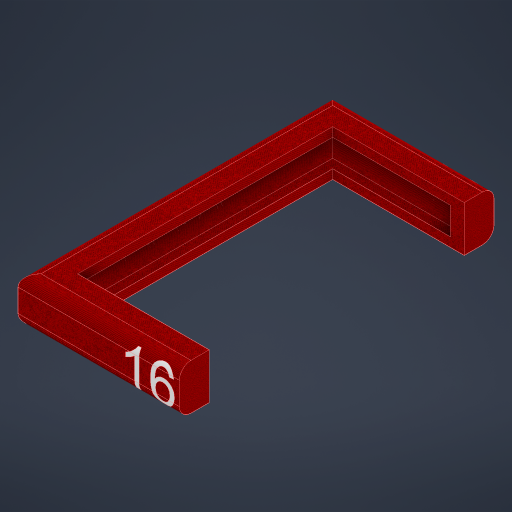
# Autodesk Inventor part: BUMP_005_BumperCloth
Saved by Autodesk Inventor 2024.2 (Build 282272000, 272)
## iProperties
Created: 2024-08-07
Part Number: BUMP_005_BumperCloth
Material: 1000 Denier Nylon Cordura
Document SubType Name: Modeling
Designer: Bryan
Density: 1 g/cm^3
Appearance: Default(1)
Mass: 229.5 g
Surface Area: 11381.8 cm^2
Volume: 229.5 cm^3
Author: Bryan
Autodesk Inventor part; units mm, degrees
ref_plane "YZ Plane" through (0, 0, 0) normal (1, 0, 0) x (0, 1, 0)
ref_plane "XZ Plane" through (0, 0, 0) normal (0, 1, 0) x (-1, 0, 0)
ref_plane "XY Plane" through (0, 0, 0) normal (0, 0, 1) x (1, 0, 0)
sketch "Sketch2" plane through (0, 0, 0) normal (1, 0, 0) x (0, 1, 0)
  line L0 (127, 0) -> (127, -82.55) construction
  line L1 (127, -82.55) -> (0, -82.55) construction
  line L2 (0, -82.55) -> (0, 0) construction
  circle A0 centre (95.25, -50.8) radius 31.75 construction
  circle A1 centre (31.75, -50.8) radius 31.75 construction
  arc A2 (95.25, -82.55) -> (127, -50.8) centre (95.25, -50.8) ccw
  arc A3 (0, -50.8) -> (31.75, -82.55) centre (31.75, -50.8) ccw
  line L3 (31.75, -82.55) -> (95.25, -82.55)
  line L4 (0, -50.8) -> (0, 0)
  line L5 (127, -50.8) -> (127, 0)
  line L6 (127, 0) -> (101.6, 0)
  line L7 (0, 0) -> (25.4, 0)
  line L8 (101.6, 0.4) -> (127.4, 0.4)
  line L9 (127.4, 0.4) -> (127.4, -50.8)
  arc A4 (95.25, -82.95) -> (127.4, -50.8) centre (95.25, -50.8) ccw
  line L10 (95.25, -82.95) -> (31.75, -82.95)
  arc A5 (-0.4, -50.8) -> (31.75, -82.95) centre (31.75, -50.8) ccw
  line L11 (-0.4, -50.8) -> (-0.4, 0.4)
  line L12 (-0.4, 0.4) -> (25.4, 0.4)
  line L13 (127, 0) -> (0, -82.55) construction
  line L14 (0, 0) -> (127, -82.55) construction
  line L15 (101.6, 0.4) -> (101.6, 0)
  line L16 (25.4, 0.4) -> (25.4, 0)
  point P0 (63.5, -41.275)
  dimension "d1" = 82.55
  dimension "d2" = 127
  dimension "d3" = 63.5
  dimension "d4" = 25.4
  dimension "d5" = 25.4
  dimension "d6" = 127
  dimension "d7" = 0.4
  constraints: 34 end point, 12 point on circle, 7 tangent, 6 centre point, 4 point on line, 4 vertical, 3 concentric, 3 horizontal, 1 equal radius, 1 midpoint, 1 parallel, 6 other
  measures "d1" distance of L0.start L0.end
  measures "d2" distance of L2.end L0.start
  measures "d3" diameter of A0
  measures "d4" distance of L0.start L6.end
  measures "d5" distance of L2.end L7.end
  measures "d6" distance of L0.end L1.end
  measures "d7" distance between parallel lines of L6 L8
sketch3d "3D Sketch1"
  line L0 (0, 63.5, -41.275) -> (-407.9875, 63.5, -41.275)
  line L1 (-407.9875, 63.5, -41.275) -> (-407.9875, 63.5, 752.475)
  line L2 (-407.9875, 63.5, 752.475) -> (0, 63.5, 752.475)
  dimension "d10" = 407.9875
  dimension "d11" = 793.75
sweep "Sweep1" add profiles "Sketch2" path "3D Sketch1"
sketch "Sketch3" plane through (0, 31.75, 793.75) normal (1, 0, 0) x (0, 0, -1)
  line L0 (793.75, -31.75) -> (793.75, -6.35) projected
  line L1 (793.75, -6.35) -> (793.35, -6.35) projected
  line L2 (793.35, -6.35) -> (793.35, -32.15) projected
  line L3 (793.35, -32.15) -> (844.55, -32.15) projected
  arc A0 (844.55, -32.15) -> (876.7, 0) centre (844.55, 0) ccw projected
  line L4 (876.7, 0) -> (876.7, 63.5) projected
  arc A1 (876.7, 63.5) -> (844.55, 95.65) centre (844.55, 63.5) ccw projected
  line L5 (844.55, 95.65) -> (793.35, 95.65) projected
  line L6 (793.35, 95.65) -> (793.35, 69.85) projected
  line L7 (793.35, 69.85) -> (793.75, 69.85) projected
  line L8 (793.75, 69.85) -> (793.75, 95.25) projected
  line L9 (793.75, 95.25) -> (844.55, 95.25) projected
  arc A2 (876.3, 63.5) -> (844.55, 95.25) centre (844.55, 63.5) ccw projected
  line L10 (876.3, 63.5) -> (876.3, 0) projected
  arc A3 (844.55, -31.75) -> (876.3, 0) centre (844.55, 0) ccw projected
  line L11 (844.55, -31.75) -> (793.75, -31.75) projected
  line L12 (793.35, 69.85) -> (793.35, -6.35)
  line L13 (82.55, -6.35) -> (82.55, -31.75) projected
  line L14 (82.55, -31.75) -> (31.75, -31.75) projected
  arc A4 (0, 0) -> (31.75, -31.75) centre (31.75, 0) ccw projected
  line L15 (0, 0) -> (0, 63.5) projected
  arc A5 (31.75, 95.25) -> (0, 63.5) centre (31.75, 63.5) ccw projected
  line L16 (31.75, 95.25) -> (82.55, 95.25) projected
  line L17 (82.55, 95.25) -> (82.55, 69.85) projected
  line L18 (82.55, 69.85) -> (82.95, 69.85) projected
  line L19 (82.95, 69.85) -> (82.95, 95.65) projected
  line L20 (82.95, 95.65) -> (31.75, 95.65) projected
  arc A6 (31.75, 95.65) -> (-0.4, 63.5) centre (31.75, 63.5) ccw projected
  line L21 (-0.4, 63.5) -> (-0.4, 0) projected
  arc A7 (-0.4, 0) -> (31.75, -32.15) centre (31.75, 0) ccw projected
  line L22 (31.75, -32.15) -> (82.95, -32.15) projected
  line L23 (82.95, -32.15) -> (82.95, -6.35) projected
  line L24 (82.95, -6.35) -> (82.55, -6.35) projected
  line L25 (82.95, 69.85) -> (82.95, -6.35)
  constraints: 4 end point, 2 vertical
extrude "Extrusion1" add sketch "Sketch3" along normal blind 0.4
sketch "Sketch4" plane through (-366.3125, 101.6, 710.8) normal (0, 0, -1) x (-1, 0, 0)
  line L0 (0, 0) -> (-366.3125, 0) projected
  line L1 (-366.3125, -76.2) -> (-366.3125, 0) projected
  line L2 (0, -76.2) -> (-366.3125, -76.2) projected
  line L3 (-328.2125, 0) -> (-328.2125, -76.2)
  point P0 (-366.3125, -101.6)
  dimension "d16" = 38.1
  constraints: 2 end point, 2 point on line, 1 vertical
  measures "d16" distance between parallel lines of L1 L3
extrude "Extrusion2" add sketch "Sketch4" against normal blind 0.4
sketch "Sketch6" plane through (0, 31.75, 793.75) normal (1, 0, 0) x (0, 0, -1)
  line L0 (82.95, 95.65) -> (31.75, 95.65) projected
  arc A0 (31.75, 95.65) -> (-0.4, 63.5) centre (31.75, 63.5) ccw construction
  line L1 (-0.4, 63.5) -> (-0.4, 0) projected
  arc A1 (-0.4, 0) -> (31.75, -32.15) centre (31.75, 0) ccw projected
  line L2 (31.75, -32.15) -> (82.95, -32.15) projected
  line L3 (82.95, -32.15) -> (82.95, 95.65) projected
  arc A2 (31.75, 95.75) -> (-0.5, 63.5) centre (31.75, 63.5) ccw
  line L4 (31.75, 95.75) -> (83.05, 95.75)
  line L5 (83.05, 95.75) -> (83.05, -32.25)
  line L6 (83.05, -32.25) -> (31.75, -32.25)
  arc A3 (-0.5, 0) -> (31.75, -32.25) centre (31.75, 0) ccw
  line L7 (-0.5, 0) -> (-0.5, 63.5)
  arc A4 (31.75, 146.55) -> (-51.3, 63.5) centre (31.75, 63.5) ccw
  line L8 (31.75, 146.55) -> (133.85, 146.55)
  line L9 (133.85, 146.55) -> (133.85, -83.05)
  line L10 (133.85, -83.05) -> (31.75, -83.05)
  arc A5 (-51.3, 0) -> (31.75, -83.05) centre (31.75, 0) ccw
  line L11 (-51.3, 0) -> (-51.3, 63.5)
  point P0 (793.75, -31.75)
  dimension "d22" = 0.1
  dimension "d51" = 50.8
  constraints: 16 end point, 8 point on circle, 4 centre point, 10 other
  measures "d22" radial gap between concentric circles of A0 A2
  measures "d51" radial gap between concentric circles of A2 A4
ref_plane "Work Plane1" through (-449.6625, 31.75, 794.25) normal (0, 0, 1) x (1, 0, 0)
sketch "Sketch5" plane through (-366.3125, -0.4, 0.4) normal (0, 0, 1) x (1, 0, 0)
  line L0 (366.3125, 102) -> (0, 102) projected
  line L1 (366.3125, 102) -> (366.3125, 25.8) projected
  line L2 (366.3125, 25.8) -> (0, 25.8) projected
  line L3 (328.2125, 102) -> (328.2125, 25.8)
  point P0 (366.3125, 0.4)
  dimension "d19" = 38.1
  constraints: 2 end point, 2 point on line, 1 vertical
  measures "d19" distance between parallel lines of L1 L3
extrude "Extrusion3" add sketch "Sketch5" against normal blind 0.4
sketch "Sketch9" plane through (-449.6625, 31.75, 794.25) normal (0, 0, 1) x (1, 0, 0)
  line L0 (284.9625, 82.95) -> (437.3625, 82.95) construction
  line L1 (437.3625, 82.95) -> (437.3625, -18.65) construction
  line L2 (437.3625, -18.65) -> (284.9625, -18.65) construction
  line L3 (284.9625, -18.65) -> (284.9625, 82.95) construction
  line L4 (32.15, 95.65) -> (450.0625, 95.65) projected
  line L5 (450.0625, 63.5) -> (450.0625, 0) projected
  line L6 (337.7759, -19.0372) -> (325.3082, -19.0372)
  line L7 (325.3082, -19.0372) -> (325.3082, 60.4152)
  spline S0 degree 2 poles (325.3082, 60.4152) (320.8168, 56.1561) (306.1808, 47.5604) (300.3729, 45.3921) knots 0 0 0 1 2 2 2
  line L8 (300.3729, 45.3921) -> (300.3729, 57.4726)
  spline S1 degree 2 poles (300.3729, 57.4726) (310.8271, 62.3512) (326.4698, 76.3677) (329.7223, 82.95) knots 0 0 0 1 2 2 2
  line L9 (329.7223, 82.95) -> (337.7759, 82.95)
  line L10 (337.7759, 82.95) -> (337.7759, -19.0372)
  line L11 (434.5747, 57.6274) -> (422.1844, 56.6207)
  spline S2 degree 2 poles (422.1844, 56.6207) (420.4808, 63.9774) (417.4607, 67.3848) knots 0 0 0 1 1 1
  spline S3 degree 2 poles (417.4607, 67.3848) (412.3497, 72.728) (404.9155, 72.728) knots 0 0 0 1 1 1
  spline S4 degree 2 poles (404.9155, 72.728) (398.9527, 72.728) (394.4613, 69.3982) knots 0 0 0 1 1 1
  spline S5 degree 2 poles (394.4613, 69.3982) (388.5759, 65.139) (381.7613, 48.5671) (381.6064, 33.3116) knots 0 0 0 1 2 2 2
  spline S6 degree 2 poles (381.6064, 33.3116) (386.0979, 40.2037) (399.1851, 46.8634) (406.3094, 46.8634) knots 0 0 0 1 2 2 2
  spline S7 degree 2 poles (406.3094, 46.8634) (418.7771, 46.8634) (436.3558, 28.5104) (436.3558, 13.9518) knots 0 0 0 1 2 2 2
  spline S8 degree 2 poles (436.3558, 13.9518) (436.3558, 4.4268) (428.0698, -11.9902) (413.6662, -20.7409) (404.5284, -20.7409) knots 0 0 0 1 2 3 3 3
  spline S9 degree 2 poles (404.5284, -20.7409) (388.8857, -20.7409) (369.2162, 2.1811) (369.2162, 28.5104) knots 0 0 0 1 2 2 2
  spline S10 degree 2 poles (369.2162, 28.5104) (369.2162, 57.9372) (380.1351, 71.3341) knots 0 0 0 1 1 1
  spline S11 degree 2 poles (380.1351, 71.3341) (389.5826, 82.95) (405.6899, 82.95) knots 0 0 0 1 1 1
  spline S12 degree 2 poles (405.6899, 82.95) (417.693, 82.95) (433.0259, 69.4756) (434.5747, 57.6274) knots 0 0 0 1 2 2 2
  spline S13 degree 2 poles (383.5424, 13.8744) (383.5424, 7.4469) (389.0405, -4.3238) (398.7979, -10.5189) (404.2186, -10.5189) knots 0 0 0 1 2 3 3 3
  spline S14 degree 2 poles (404.2186, -10.5189) (412.1948, -10.5189) (423.5009, 2.2585) (423.5009, 13.1774) knots 0 0 0 1 2 2 2
  spline S15 degree 2 poles (423.5009, 13.1774) (423.5009, 23.7091) (412.3497, 35.8671) (403.754, 35.8671) knots 0 0 0 1 2 2 2
  spline S16 degree 2 poles (403.754, 35.8671) (395.3131, 35.8671) (383.5424, 23.7091) (383.5424, 13.8744) knots 0 0 0 1 2 2 2
  point P0 (449.6625, -31.75)
  dimension "d31" = 101.6
  dimension "d32" = 152.4
  dimension "d33" = 12.7
  dimension "d34" = 12.7
  constraints: 2 other
  measures "d31" distance of L0.end L1.end
  measures "d32" distance of L0.start L0.end
  measures "d33" distance between parallel lines of L4 L0
  measures "d34" distance between parallel lines of L5 L1
extrude "Extrusion4" add sketch "Sketch9" against normal blind 12.7
ref_plane "Work Plane2" through (-449.7625, 31.75, -82.95) normal (-1, 0, 0) x (0, 0, 1)
sketch "Sketch10" plane through (-449.7625, 31.75, -82.95) normal (-1, 0, 0) x (0, 0, 1)
  line L0 (273.45, 82.15) -> (603.65, 82.15) construction
  line L1 (603.65, 82.15) -> (603.65, -19.45) construction
  line L2 (603.65, -19.45) -> (273.45, -19.45) construction
  line L3 (273.45, -19.45) -> (273.45, 82.15) construction
  line L4 (32.15, -32.15) -> (844.95, -32.15) projected
  line L5 (0, 63.5) -> (0, 0) projected
  line L6 (877.1, 63.5) -> (877.1, 0) projected
  line L7 (326.2634, -19.8372) -> (313.7957, -19.8372)
  line L8 (313.7957, -19.8372) -> (313.7957, 59.6152)
  spline S0 degree 2 poles (313.7957, 59.6152) (309.3043, 55.3561) (294.6683, 46.7604) (288.8604, 44.5921) knots 0 0 0 1 2 2 2
  line L9 (288.8604, 44.5921) -> (288.8604, 56.6726)
  spline S1 degree 2 poles (288.8604, 56.6726) (299.3146, 61.5512) (314.9573, 75.5677) (318.2098, 82.15) knots 0 0 0 1 2 2 2
  line L10 (318.2098, 82.15) -> (326.2634, 82.15)
  line L11 (326.2634, 82.15) -> (326.2634, -19.8372)
  line L12 (423.0622, 56.8274) -> (410.6719, 55.8207)
  spline S2 degree 2 poles (410.6719, 55.8207) (408.9683, 63.1774) (405.9482, 66.5848) knots 0 0 0 1 1 1
  spline S3 degree 2 poles (405.9482, 66.5848) (400.8372, 71.928) (393.403, 71.928) knots 0 0 0 1 1 1
  spline S4 degree 2 poles (393.403, 71.928) (387.4402, 71.928) (382.9488, 68.5982) knots 0 0 0 1 1 1
  spline S5 degree 2 poles (382.9488, 68.5982) (377.0634, 64.339) (370.2488, 47.7671) (370.0939, 32.5116) knots 0 0 0 1 2 2 2
  spline S6 degree 2 poles (370.0939, 32.5116) (374.5854, 39.4037) (387.6726, 46.0634) (394.7969, 46.0634) knots 0 0 0 1 2 2 2
  spline S7 degree 2 poles (394.7969, 46.0634) (407.2646, 46.0634) (424.8433, 27.7104) (424.8433, 13.1518) knots 0 0 0 1 2 2 2
  spline S8 degree 2 poles (424.8433, 13.1518) (424.8433, 3.6268) (416.5573, -12.7902) (402.1537, -21.5409) (393.0159, -21.5409) knots 0 0 0 1 2 3 3 3
  spline S9 degree 2 poles (393.0159, -21.5409) (377.3732, -21.5409) (357.7037, 1.3811) (357.7037, 27.7104) knots 0 0 0 1 2 2 2
  spline S10 degree 2 poles (357.7037, 27.7104) (357.7037, 57.1372) (368.6226, 70.5341) knots 0 0 0 1 1 1
  spline S11 degree 2 poles (368.6226, 70.5341) (378.0701, 82.15) (394.1774, 82.15) knots 0 0 0 1 1 1
  spline S12 degree 2 poles (394.1774, 82.15) (406.1805, 82.15) (421.5134, 68.6756) (423.0622, 56.8274) knots 0 0 0 1 2 2 2
  spline S13 degree 2 poles (372.0299, 13.0744) (372.0299, 6.6469) (377.528, -5.1238) (387.2854, -11.3189) (392.7061, -11.3189) knots 0 0 0 1 2 3 3 3
  spline S14 degree 2 poles (392.7061, -11.3189) (400.6823, -11.3189) (411.9884, 1.4585) (411.9884, 12.3774) knots 0 0 0 1 2 2 2
  spline S15 degree 2 poles (411.9884, 12.3774) (411.9884, 22.9091) (400.8372, 35.0671) (392.2415, 35.0671) knots 0 0 0 1 2 2 2
  spline S16 degree 2 poles (392.2415, 35.0671) (383.8006, 35.0671) (372.0299, 22.9091) (372.0299, 13.0744) knots 0 0 0 1 2 2 2
  line L13 (502.6695, -7.8342) -> (502.6695, -19.8372)
  line L14 (502.6695, -19.8372) -> (435.5299, -19.8372)
  spline S17 degree 2 poles (435.5299, -19.8372) (435.375, -15.3457) (437.0012, -11.164) knots 0 0 0 1 1 1
  spline S18 degree 2 poles (437.0012, -11.164) (439.5567, -4.272) (450.8628, 8.9701) (461.5494, 17.7207) knots 0 0 0 1 2 2 2
  spline S19 degree 2 poles (461.5494, 17.7207) (478.0439, 31.35) (489.6598, 47.1476) (489.6598, 54.2719) knots 0 0 0 1 2 2 2
  spline S20 degree 2 poles (489.6598, 54.2719) (489.6598, 61.7061) (479.0506, 71.8506) (470.5323, 71.8506) knots 0 0 0 1 2 2 2
  spline S21 degree 2 poles (470.5323, 71.8506) (461.5494, 71.8506) (450.7854, 61.0091) (450.7079, 51.4841) knots 0 0 0 1 2 2 2
  line L15 (450.7079, 51.4841) -> (437.853, 52.8006)
  spline S22 degree 2 poles (437.853, 52.8006) (439.1695, 67.1268) (456.361, 82.15) (470.8421, 82.15) knots 0 0 0 1 2 2 2
  spline S23 degree 2 poles (470.8421, 82.15) (485.478, 82.15) (502.5146, 65.9652) (502.5146, 53.9622) knots 0 0 0 1 2 2 2
  spline S24 degree 2 poles (502.5146, 53.9622) (502.5146, 47.8445) (497.5585, 36.0738) (485.9427, 23.064) (472.5457, 11.6805) knots 0 0 0 1 2 3 3 3
  spline S25 degree 2 poles (472.5457, 11.6805) (461.3171, 2.3104) (454.9671, -4.4268) (452.8762, -7.8342) knots 0 0 0 1 2 2 2
  line L16 (452.8762, -7.8342) -> (502.6695, -7.8342)
  line L17 (581.5799, -7.8342) -> (581.5799, -19.8372)
  line L18 (581.5799, -19.8372) -> (514.4402, -19.8372)
  spline S26 degree 2 poles (514.4402, -19.8372) (514.2854, -15.3457) (515.9116, -11.164) knots 0 0 0 1 1 1
  spline S27 degree 2 poles (515.9116, -11.164) (518.4671, -4.272) (529.7732, 8.9701) (540.4598, 17.7207) knots 0 0 0 1 2 2 2
  spline S28 degree 2 poles (540.4598, 17.7207) (556.9543, 31.35) (568.5701, 47.1476) (568.5701, 54.2719) knots 0 0 0 1 2 2 2
  spline S29 degree 2 poles (568.5701, 54.2719) (568.5701, 61.7061) (557.961, 71.8506) (549.4427, 71.8506) knots 0 0 0 1 2 2 2
  spline S30 degree 2 poles (549.4427, 71.8506) (540.4598, 71.8506) (529.6957, 61.0091) (529.6183, 51.4841) knots 0 0 0 1 2 2 2
  line L19 (529.6183, 51.4841) -> (516.7634, 52.8006)
  spline S31 degree 2 poles (516.7634, 52.8006) (518.0799, 67.1268) (535.2713, 82.15) (549.7524, 82.15) knots 0 0 0 1 2 2 2
  spline S32 degree 2 poles (549.7524, 82.15) (564.3884, 82.15) (581.425, 65.9652) (581.425, 53.9622) knots 0 0 0 1 2 2 2
  spline S33 degree 2 poles (581.425, 53.9622) (581.425, 47.8445) (576.4689, 36.0738) (564.853, 23.064) (551.4561, 11.6805) knots 0 0 0 1 2 3 3 3
  spline S34 degree 2 poles (551.4561, 11.6805) (540.2274, 2.3104) (533.8774, -4.4268) (531.7866, -7.8342) knots 0 0 0 1 2 2 2
  line L20 (531.7866, -7.8342) -> (581.5799, -7.8342)
  point P0 (82.95, -31.75)
  point P1 (438.55, 82.15)
  dimension "d38" = 330.2
  dimension "d39" = 101.6
  dimension "d40" = 12.7
  dimension "d41" = 438.55
  dimension "d56" = 877.1
  constraints: 1 midpoint, 2 other
  measures "d38" distance of L0.start L0.end
  measures "d39" distance of L2.end L0.start
  measures "d40" distance between parallel lines of L4 L2
  measures "d41" distance from line of L5 point (438.55, 82.15)
  measures "d56" distance between parallel lines of L6 L5
extrude "Extrusion5" add sketch "Sketch10" against normal blind 12.7
ref_plane "Work Plane3" through (-449.6625, 31.75, -83.05) normal (0, 0, -1) x (-1, 0, 0)
sketch "Sketch11" plane through (-449.6625, 31.75, -83.05) normal (0, 0, -1) x (-1, 0, 0)
  line L0 (-437.3625, 82.55) -> (-284.9625, 82.55) construction
  line L1 (-284.9625, 82.55) -> (-284.9625, -19.05) construction
  line L2 (-284.9625, -19.05) -> (-437.3625, -19.05) construction
  line L3 (-437.3625, -19.05) -> (-437.3625, 82.55) construction
  line L4 (-449.6625, 95.25) -> (-32.15, 95.25) projected
  line L5 (-450.0625, 0) -> (-450.0625, 63.5) projected
  line L6 (-365.9637, -7.4342) -> (-365.9637, -19.4372)
  line L7 (-365.9637, -19.4372) -> (-433.1034, -19.4372)
  spline S0 degree 2 poles (-433.1034, -19.4372) (-433.2582, -14.9457) (-431.632, -10.764) knots 0 0 0 1 1 1
  spline S1 degree 2 poles (-431.632, -10.764) (-429.0765, -3.872) (-417.7704, 9.3701) (-407.0838, 18.1207) knots 0 0 0 1 2 2 2
  spline S2 degree 2 poles (-407.0838, 18.1207) (-390.5893, 31.75) (-378.9735, 47.5476) (-378.9735, 54.6719) knots 0 0 0 1 2 2 2
  spline S3 degree 2 poles (-378.9735, 54.6719) (-378.9735, 62.1061) (-389.5826, 72.2506) (-398.1009, 72.2506) knots 0 0 0 1 2 2 2
  spline S4 degree 2 poles (-398.1009, 72.2506) (-407.0838, 72.2506) (-417.8479, 61.4091) (-417.9253, 51.8841) knots 0 0 0 1 2 2 2
  line L8 (-417.9253, 51.8841) -> (-430.7802, 53.2006)
  spline S5 degree 2 poles (-430.7802, 53.2006) (-429.4637, 67.5268) (-412.2723, 82.55) (-397.7912, 82.55) knots 0 0 0 1 2 2 2
  spline S6 degree 2 poles (-397.7912, 82.55) (-383.1552, 82.55) (-366.1186, 66.3652) (-366.1186, 54.3622) knots 0 0 0 1 2 2 2
  spline S7 degree 2 poles (-366.1186, 54.3622) (-366.1186, 48.2445) (-371.0747, 36.4738) (-382.6905, 23.464) (-396.0875, 12.0805) knots 0 0 0 1 2 3 3 3
  spline S8 degree 2 poles (-396.0875, 12.0805) (-407.3162, 2.7104) (-413.6662, -4.0268) (-415.757, -7.4342) knots 0 0 0 1 2 2 2
  line L9 (-415.757, -7.4342) -> (-365.9637, -7.4342)
  line L10 (-287.0534, -7.4342) -> (-287.0534, -19.4372)
  line L11 (-287.0534, -19.4372) -> (-354.193, -19.4372)
  spline S9 degree 2 poles (-354.193, -19.4372) (-354.3479, -14.9457) (-352.7216, -10.764) knots 0 0 0 1 1 1
  spline S10 degree 2 poles (-352.7216, -10.764) (-350.1662, -3.872) (-338.8601, 9.3701) (-328.1735, 18.1207) knots 0 0 0 1 2 2 2
  spline S11 degree 2 poles (-328.1735, 18.1207) (-311.679, 31.75) (-300.0631, 47.5476) (-300.0631, 54.6719) knots 0 0 0 1 2 2 2
  spline S12 degree 2 poles (-300.0631, 54.6719) (-300.0631, 62.1061) (-310.6723, 72.2506) (-319.1906, 72.2506) knots 0 0 0 1 2 2 2
  spline S13 degree 2 poles (-319.1906, 72.2506) (-328.1735, 72.2506) (-338.9375, 61.4091) (-339.0149, 51.8841) knots 0 0 0 1 2 2 2
  line L12 (-339.0149, 51.8841) -> (-351.8698, 53.2006)
  spline S14 degree 2 poles (-351.8698, 53.2006) (-350.5534, 67.5268) (-333.3619, 82.55) (-318.8808, 82.55) knots 0 0 0 1 2 2 2
  spline S15 degree 2 poles (-318.8808, 82.55) (-304.2448, 82.55) (-287.2082, 66.3652) (-287.2082, 54.3622) knots 0 0 0 1 2 2 2
  spline S16 degree 2 poles (-287.2082, 54.3622) (-287.2082, 48.2445) (-292.1643, 36.4738) (-303.7802, 23.464) (-317.1771, 12.0805) knots 0 0 0 1 2 3 3 3
  spline S17 degree 2 poles (-317.1771, 12.0805) (-328.4058, 2.7104) (-334.7558, -4.0268) (-336.8466, -7.4342) knots 0 0 0 1 2 2 2
  line L13 (-336.8466, -7.4342) -> (-287.0534, -7.4342)
  point P0 (-449.6625, -31.75)
  dimension "d45" = 152.4
  dimension "d46" = 101.6
  dimension "d47" = 12.7
  dimension "d48" = 12.7
  constraints: 2 other
  measures "d45" distance of L0.start L0.end
  measures "d46" distance of L0.end L1.end
  measures "d47" distance between parallel lines of L4 L0
  measures "d48" distance between parallel lines of L3 L5
extrude "Extrusion6" add sketch "Sketch11" against normal blind 12.7
sketch3d "3D Sketch1 for Sweep2"
  line L0 (0, 63.5, 752.475) -> (-407.9875, 63.5, 752.475)
  line L1 (-407.9875, 63.5, 752.475) -> (-407.9875, 63.5, -41.275)
  line L2 (-407.9875, 63.5, -41.275) -> (0, 63.5, -41.275)
  dimension "d10" = 407.9875
  dimension "d11" = 793.75
sweep "Sweep2" cut profiles "Sketch6" path "3D Sketch1 for Sweep2"
sketch "Sketch12" plane through (0, 31.75, 793.75) normal (-1, 0, 0) x (0, 0, 1)
  line L0 (-793.75, -31.75) -> (-793.75, 95.25) projected
  line L1 (-793.75, 95.25) -> (-844.55, 95.25) projected
  arc A0 (-844.55, 95.25) -> (-876.3, 63.5) centre (-844.55, 63.5) ccw projected
  line L2 (-876.3, 63.5) -> (-876.3, 0) projected
  arc A1 (-876.3, 0) -> (-844.55, -31.75) centre (-844.55, 0) ccw projected
  line L3 (-844.55, -31.75) -> (-793.75, -31.75) projected
sketch3d "3D Sketch1 for Sweep3"
  line L0 (0, 63.5, -41.275) -> (-407.9875, 63.5, -41.275)
  line L1 (-407.9875, 63.5, -41.275) -> (-407.9875, 63.5, 752.475)
  line L2 (-407.9875, 63.5, 752.475) -> (0, 63.5, 752.475)
  dimension "d10" = 407.9875
  dimension "d11" = 793.75
sweep "Sweep3" cut profiles "Sketch12" path "3D Sketch1 for Sweep3"
equation "\"d41\" = 0.5 * d56"
body "Solid1"
